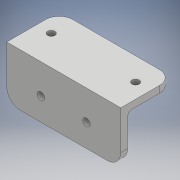
# Autodesk Inventor part: FrontIRHolder
Saved by Autodesk Inventor 2018 (Build 220112000, 112)
## iProperties
Created: 2018-05-03
Part Number: FrontIRHolder
Material: Generic
Document SubType Name: Modeling
Designer: alexs
Density: 1 g/cm^3
Appearance: Default
Author: alexs
Autodesk Inventor part; units mm, degrees
ref_plane "YZ Plane" through (0, 0, 0) normal (1, 0, 0) x (0, 1, 0)
ref_plane "XZ Plane" through (0, 0, 0) normal (0, 1, 0) x (-1, 0, 0)
ref_plane "XY Plane" through (0, 0, 0) normal (0, 0, 1) x (1, 0, 0)
sketch "Sketch1" plane through (0, 0, 0) normal (0, 1, 0) x (-1, 0, 0)
  line L0 (0, 0) -> (-50, 0)
  line L1 (-50, 0) -> (-50, -23)
  line L2 (-50, -23) -> (0, -23)
  line L3 (0, -23) -> (0, 0)
  dimension "d0" = 50
  dimension "d1" = 23
  constraints: 8 end point, 2 parallel, 1 horizontal, 1 perpendicular
  measures "d0" distance of L2.end L1.end
  measures "d1" distance of L1.end L0.end
extrude "Extrusion1" add sketch "Sketch1" along normal blind 3
sketch "Sketch2" plane through (0, 3, 0) normal (0, 1, 0) x (1, 0, 0)
  line L0 (0, 23) -> (0, 0) construction
  line L1 (0, 0) -> (50, 0) construction
  line L2 (50, 0) -> (50, 23) construction
  line L3 (0, 3) -> (50, 3)
  line L4 (50, 3) -> (50, 0)
  line L5 (50, 0) -> (0, 0)
  line L6 (0, 0) -> (0, 3)
  dimension "d4" = 3
  constraints: 8 end point, 2 parallel, 1 horizontal, 1 perpendicular, 1 point on line
  measures "d4" distance between parallel lines of L1 L3
extrude "Extrusion2" add sketch "Sketch2" along normal blind 20
sketch "Sketch3" plane through (0, 0, 0) normal (0, 0, 1) x (1, 0, 0)
  circle A0 centre (6.5, 13) radius 1.6
  circle A1 centre (43.5, 13) radius 1.6
  line L0 (0, 0) -> (0, 23) projected
  line L1 (0, 23) -> (50, 23) projected
  dimension "d7" = 3.2
  dimension "d8" = 3.2
  dimension "d9" = 37
  dimension "d10" = 6.5
  dimension "d11" = 10
  dimension "d12" = 10
  constraints: 2 centre point
  measures "d7" diameter of A0
  measures "d8" diameter of A1
  measures "d9" distance of A0.centre A1.centre
  measures "d10" distance from line of L0 A0.centre
  measures "d11" distance from line of L1 A0.centre
  measures "d12" distance from line of L1 A1.centre
extrude "Extrusion3" cut sketch "Sketch3" against normal through all
fillet "Fillet1" radius 6 4 edges at (0, 23, -1.5) (50, 23, -1.5) (0, 1.5, -23) (50, 1.5, -23)
fillet "Fillet2" radius 2 1 edges at (25, 3, -3)
sketch "Sketch4" plane through (0, 3, 0) normal (0, 1, 0) x (1, 0, 0)
  circle A0 centre (35, 13) radius 1.6
  circle A1 centre (15, 13) radius 1.6
  line L0 (44, 23) -> (6, 23) projected
  line L1 (50, 5) -> (50, 17) projected
  point P0 (0, 0)
  dimension "d17" = 3.2
  dimension "d18" = 3.2
  dimension "d19" = 10
  dimension "d20" = 20
  dimension "d21" = 15
  constraints: 2 centre point, 1 horizontal alignment
  measures "d17" diameter of A0
  measures "d18" diameter of A1
  measures "d19" distance from line of L0 A0.centre
  measures "d20" distance of A1.centre A0.centre
  measures "d21" distance from line of L1 A0.centre
extrude "Extrusion4" cut sketch "Sketch4" against normal through all
equation "\"d8\" = d7"
equation "\"d12\" = d11"
body "Solid1"
